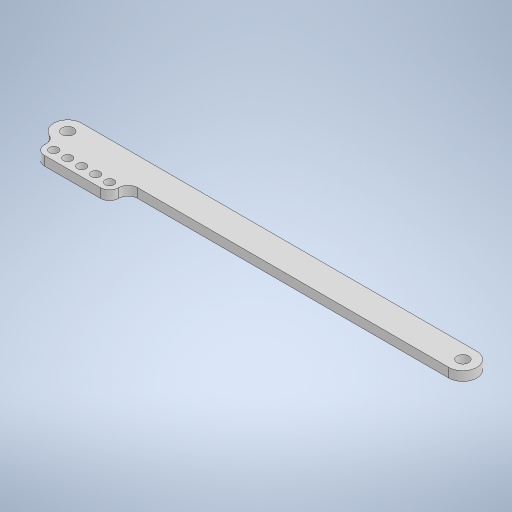
# Autodesk Inventor part: Wind Tool
Saved by Autodesk Inventor 2023.2 (Build 272271000, 271)
## iProperties
Created: 2024-03-03
Part Number: Wind Tool
Material: Generic
Document SubType Name: Modeling
Designer: Nathan Cai
Density: 1 g/cm^3
Appearance: Default
Author: Nathan Cai
Autodesk Inventor part; units mm, degrees
ref_plane "YZ Plane" through (0, 0, 0) normal (1, 0, 0) x (0, 1, 0)
ref_plane "XZ Plane" through (0, 0, 0) normal (0, 1, 0) x (-1, 0, 0)
ref_plane "XY Plane" through (0, 0, 0) normal (0, 0, 1) x (1, 0, 0)
sketch "Sketch1" plane through (0, 0, 0) normal (0, 1, 0) x (-1, 0, 0)
  line L0 (0, 0) -> (-134.9375, 0) construction
  line L1 (0, 4.7625) -> (-134.9375, 4.7625)
  line L2 (-134.9375, -4.7625) -> (0, -4.7625)
  arc A0 (0, -4.7625) -> (0, 4.7625) centre (0, 0) ccw
  arc A1 (-134.9375, 4.7625) -> (-134.9375, -4.7625) centre (-134.9375, 0) ccw
  circle A2 centre (0, 0) radius 2
  circle A3 centre (-134.9375, 0) radius 2
  line L3 (0, 4.7625) -> (-25.4, 4.7625)
  line L4 (-25.4, 4.7625) -> (-25.4, 11.1125)
  line L5 (-25.4, 11.1125) -> (0, 11.1125)
  line L6 (0, 11.1125) -> (0, 4.7625)
  line L7 (-25.4, 7.9375) -> (0, 7.9375) construction
  circle A4 centre (-22.225, 7.9375) radius 1.5
  circle A5 centre (-17.4625, 7.9375) radius 1.5
  circle A6 centre (-12.7, 7.9375) radius 1.5
  circle A7 centre (-7.9375, 7.9375) radius 1.5
  circle A8 centre (-3.175, 7.9375) radius 1.5
  point P0 (-67.4688, 0)
  dimension "d0" = 134.9375
  dimension "d1" = 9.525
  dimension "d2" = 4
  dimension "d3" = 4
  dimension "d6" = 25.4
  dimension "d7" = 6.35
  dimension "d8" = 3
  dimension "d9" = 3.175
  dimension "d12" = 4.7625
  constraints: 18 end point, 9 centre point, 4 point on circle, 4 tangent, 3 horizontal, 3 midpoint, 3 parallel, 2 coincident, 1 perpendicular, 1 point on line, 8 other
  measures "d0" distance of L0.start L0.end
  measures "d1" diameter of A1
  measures "d2" diameter of A2
  measures "d3" diameter of A3
  measures "d6" distance of L4.end L5.end
  measures "d7" distance of L3.end L4.end
  measures "d8" diameter of A4
  measures "d9" distance from line of L4 A4.centre
  measures "d12" distance of A4.centre A5.centre
extrude "Extrusion1" add sketch "Sketch1" along normal blind 3.175
fillet "Fillet1" radius 3.175 4 edges at (25.4, 1.5875, 4.7625) (25.4, 1.5875, 11.1125) (0, 1.5875, 11.1125) (0, 1.5875, 4.7625)
equation "\"d2\" = d3"
body "Solid1"
